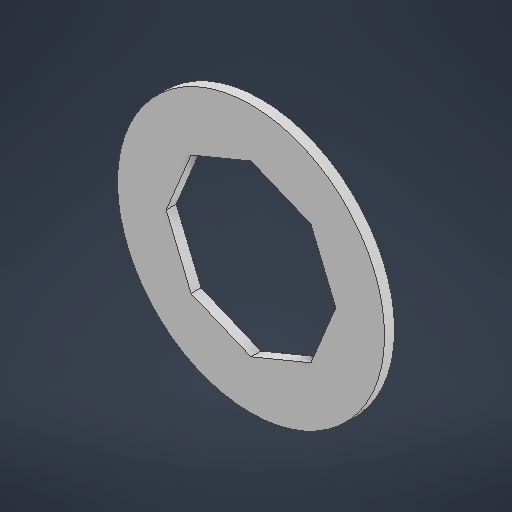
# Autodesk Inventor part: espaciador1.5mm
Saved by Autodesk Inventor 2026.1 (Build 301233020, 233B)
## iProperties
Created: 2025-11-30
Part Number: espaciador1.5mm
Material: Genérico
Document SubType Name: Modeling
Designer: TUF GAMING F15
Density: 1 g/cm^3
Appearance: Valor por defecto
Author: TUF GAMING F15
Autodesk Inventor part; units mm, degrees
ref_plane "YZ Plane" through (0, 0, 0) normal (1, 0, 0) x (0, 1, 0)
ref_plane "XZ Plane" through (0, 0, 0) normal (0, 1, 0) x (-1, 0, 0)
ref_plane "XY Plane" through (0, 0, 0) normal (0, 0, 1) x (1, 0, 0)
sketch "Boceto1" plane through (0, 0, 0) normal (0, 0, 1) x (1, 0, 0)
  circle A0 centre (0, 0) radius 20
  circle A1 centre (0, 0) radius 12.7 construction
  line L0 (0, 12.7) -> (8.9803, 8.9803)
  line L1 (8.9803, 8.9803) -> (12.7, 0)
  line L2 (12.7, 0) -> (8.9803, -8.9803)
  line L3 (8.9803, -8.9803) -> (0, -12.7)
  line L4 (0, -12.7) -> (-8.9803, -8.9803)
  line L5 (-8.9803, -8.9803) -> (-12.7, 0)
  line L6 (-12.7, 0) -> (-8.9803, 8.9803)
  line L7 (-8.9803, 8.9803) -> (0, 12.7)
  dimension "d1" = 25.4
  dimension "d0" = 40
  constraints: 16 end point, 3 coincident, 1 centre point, 1 vertical alignment, 19 other
  measures "d0" diameter of A0
extrude "Extrusión1" add sketch "Boceto1" along normal blind 1.5
